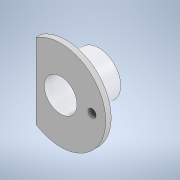
# Autodesk Inventor part: Buje de Resina
Saved by Autodesk Inventor 2020 (Build 240168000, 168)
## iProperties
Created: 2020-05-03
Part Number: Buje de Resina
Material: Acetal Resin, White
Document SubType Name: Modeling
Designer: Leon
Density: 1.425 g/cm^3
Appearance: Default
Mass: 2.35943 g
Surface Area: 19.2341 cm^2
Volume: 1.65574 cm^3
Author: Leon
Autodesk Inventor part; units mm, degrees
ref_plane "YZ Plane" through (0, 0, 0) normal (1, 0, 0) x (0, 1, 0)
ref_plane "XZ Plane" through (0, 0, 0) normal (0, 1, 0) x (-1, 0, 0)
ref_plane "XY Plane" through (0, 0, 0) normal (0, 0, 1) x (1, 0, 0)
sketch "Boceto1" plane through (0, 0, 0) normal (0, 1, 0) x (-1, 0, 0)
  line L0 (47.5409, -260.2193) -> (47.5409, -272.2193)
  line L1 (56.0409, -260.2193) -> (56.0409, -258.2193)
  line L2 (45.5409, -260.2193) -> (45.5409, -272.2193)
  line L3 (39.5409, -272.2193) -> (39.5409, -258.2193)
  line L4 (45.5409, -260.2193) -> (45.5409, -258.2193)
  line L5 (47.5409, -260.2193) -> (56.0409, -260.2193)
  line L6 (56.0409, -258.2193) -> (45.5409, -258.2193)
  line L7 (47.5409, -272.2193) -> (45.5409, -272.2193)
  dimension "d104" = 8.5
  dimension "d105" = 2
  dimension "d109" = 2
  dimension "d110" = 6
  constraints: 16 end point, 2 horizontal, 2 vertical, 1 parallel
  measures "d104" distance from line of L1.start L0
  measures "d105" distance of L1.start L1.end
  measures "d109" distance of L0.end L2.end
  measures "d110" distance between parallel lines of L3 L2
ref_plane "Work Plane1" through (-12, 0, -11) normal (0, 0, 1) x (1, 0, 0)
revolve "Revolution1" add sketch "Boceto1" angle 360 about axis through (-39.5409, 0, -272.2193) along (0, 0, 1)
sketch "Sketch5" plane through (-39.5409, 0, -258.2193) normal (0, 0, 1) x (1, 0, 0)
  circle A0 centre (0, 0) radius 8 projected
  line L0 (-9, -15.609) -> (-9, 11.134)
  circle A1 centre (0, 0) radius 16.5 projected
  line L1 (16.5, 0) -> (16.5, 3.728)
  line L2 (8, 0) -> (8, 3.728)
  circle A2 centre (11.5, 0) radius 1.5
  line L3 (13, 0) -> (13, 2.0682)
  line L4 (10, 0) -> (10, 1.5)
  line L5 (-9, 11.134) -> (-9, 14.5912)
  point P0 (39.5409, 0)
  point P1 (-9, 9.3808)
  point P2 (-9, -13.8293)
  point P3 (-9, 13.8293)
  dimension "d137" = 3
  dimension "d138" = 3.5
  constraints: 12 end point, 6 vertical, 2 point on circle, 1 centre point, 1 horizontal alignment, 3 other
  measures "d137" diameter of A2
  measures "d138" distance between parallel lines of L1 L3
extrude "Extrusion10" cut sketch "Sketch5" against normal blind 10 contours A1 L5 L0 | A2 picked at (-10.0415, -4.6289)
body "Solid2"
